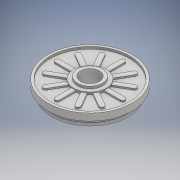
# Autodesk Inventor part: MotorGrill
Saved by Autodesk Inventor 2017 (Build 210142000, 142)
## iProperties
Created: 2017-08-24
Part Number: MotorGrill
Material: Generic
Document SubType Name: Modeling
Designer: MineV
Density: 1 g/cm^3
Appearance: Default
Author: MineV
Autodesk Inventor part; units mm, degrees
ref_plane "YZ Plane" through (0, 0, 0) normal (1, 0, 0) x (0, 1, 0)
ref_plane "XZ Plane" through (0, 0, 0) normal (0, 1, 0) x (-1, 0, 0)
ref_plane "XY Plane" through (0, 0, 0) normal (0, 0, 1) x (1, 0, 0)
sketch "Sketch1" plane through (0, 0, 0) normal (0, 1, 0) x (-1, 0, 0)
  line L0 (0, 0) -> (-27, 0)
  line L1 (-27, 0) -> (-27, -3)
  line L2 (-27, -3) -> (-22.5, -3)
  line L3 (-22.5, -3) -> (-22.5, -5.5)
  line L4 (-22.5, -5.5) -> (-24.5, -5.5)
  line L5 (-24.5, -5.5) -> (-24.5, -7.5)
  line L6 (-24.5, -7.5) -> (-20.5, -7.5)
  line L7 (-20.5, -7.5) -> (-20.5, -1.5)
  line L8 (-20.5, -1.5) -> (-8, -1.5)
  line L9 (-8, -1.5) -> (-8, -12.5)
  line L10 (-8, -12.5) -> (-6, -12.5)
  line L11 (-6, -12.5) -> (-6, 0)
  line L12 (-6, 0) -> (-6, 3)
  line L13 (-6, 3) -> (-8, 3)
  line L14 (-8, 3) -> (-8, 1.5)
  line L15 (-8, 1.5) -> (-9, 1.5)
  line L16 (-9, 1.5) -> (-10.5, 1.5)
  line L17 (-10.5, 1.5) -> (-10.5, 0)
  line L18 (-27, 0) -> (-27, 1.5)
  line L19 (-27, 1.5) -> (-25.5, 1.5)
  line L20 (-25.5, 1.5) -> (-25.5, 0)
  line L21 (0, -15.6) -> (0, 6.1) projected
  dimension "d0" = 27
  dimension "d1" = 3
  dimension "d2" = 4.5
  dimension "d3" = 2.5
  dimension "d4" = 2
  dimension "d5" = 2.5
  dimension "d6" = 4
  dimension "d7" = 2
  dimension "d8" = 1.5
  dimension "d9" = 8
  dimension "d10" = 3
  dimension "d11" = 2
  dimension "d12" = 1.5
  dimension "d13" = 1
  dimension "d14" = 1.5
  dimension "d15" = 1.5
  dimension "d16" = 5
  constraints: 42 end point, 14 perpendicular, 6 point on line, 2 horizontal, 2 vertical, 1 parallel
  measures "d0" distance of L0.start L0.end
  measures "d1" distance of L0.end L1.end
  measures "d2" distance of L1.end L2.end
  measures "d3" distance of L2.end L3.end
  measures "d4" distance of L4.end L5.end
  measures "d5" distance between parallel lines of L1 L5
  measures "d6" distance of L5.end L6.end
  measures "d7" distance of L9.end L10.end
  measures "d8" distance between parallel lines of L0 L8
  measures "d9" distance from line of L0.start L9
  measures "d10" distance of L11.end L12.end
  measures "d11" distance of L12.end L13.end
  measures "d12" distance of L13.end L14.end
  measures "d13" distance of L14.end L15.end
  measures "d14" distance of L15.end L16.end
  measures "d15" distance of L18.end L19.end
  measures "d16" distance between parallel lines of L6 L10
revolve "Revolution1" add sketch "Sketch1" angle 360 about axis through (0, 0, -10) along (0, 0, 1)
sketch "Sketch2" plane through (0, 0, 0) normal (0, 0, 1) x (1, 0, 0)
  circle A0 centre (0, 0) radius 10.5 projected
  line L0 (9.5, 1.5) -> (21, 1.5)
  line L1 (22.5, 0) -> (22.5, 0)
  line L2 (21, -1.5) -> (9.5, -1.5)
  line L3 (9.5, -1.5) -> (9.5, 1.5)
  arc A1 (22.5, 0) -> (21, 1.5) centre (21, 0) ccw
  arc A2 (21, -1.5) -> (22.5, 0) centre (21, 0) ccw
  line L4 (7.4772, 6.049) -> (17.4365, 11.799)
  line L5 (19.4856, 11.25) -> (19.4856, 11.25)
  line L6 (18.9365, 9.201) -> (8.9772, 3.451)
  line L7 (8.9772, 3.451) -> (7.4772, 6.049)
  arc A3 (19.4856, 11.25) -> (17.4365, 11.799) centre (18.1865, 10.5) ccw
  arc A4 (18.9365, 9.201) -> (19.4856, 11.25) centre (18.1865, 10.5) ccw
  line L8 (3.451, 8.9772) -> (9.201, 18.9365)
  line L9 (11.25, 19.4856) -> (11.25, 19.4856)
  line L10 (11.799, 17.4365) -> (6.049, 7.4772)
  line L11 (6.049, 7.4772) -> (3.451, 8.9772)
  arc A5 (11.25, 19.4856) -> (9.201, 18.9365) centre (10.5, 18.1865) ccw
  arc A6 (11.799, 17.4365) -> (11.25, 19.4856) centre (10.5, 18.1865) ccw
  line L12 (-1.5, 9.5) -> (-1.5, 21)
  line L13 (0, 22.5) -> (0, 22.5)
  line L14 (1.5, 21) -> (1.5, 9.5)
  line L15 (1.5, 9.5) -> (-1.5, 9.5)
  arc A7 (0, 22.5) -> (-1.5, 21) centre (0, 21) ccw
  arc A8 (1.5, 21) -> (0, 22.5) centre (0, 21) ccw
  line L16 (-6.049, 7.4772) -> (-11.799, 17.4365)
  line L17 (-11.25, 19.4856) -> (-11.25, 19.4856)
  line L18 (-9.201, 18.9365) -> (-3.451, 8.9772)
  line L19 (-3.451, 8.9772) -> (-6.049, 7.4772)
  arc A9 (-11.25, 19.4856) -> (-11.799, 17.4365) centre (-10.5, 18.1865) ccw
  arc A10 (-9.201, 18.9365) -> (-11.25, 19.4856) centre (-10.5, 18.1865) ccw
  line L20 (-8.9772, 3.451) -> (-18.9365, 9.201)
  line L21 (-19.4856, 11.25) -> (-19.4856, 11.25)
  line L22 (-17.4365, 11.799) -> (-7.4772, 6.049)
  line L23 (-7.4772, 6.049) -> (-8.9772, 3.451)
  arc A11 (-19.4856, 11.25) -> (-18.9365, 9.201) centre (-18.1865, 10.5) ccw
  arc A12 (-17.4365, 11.799) -> (-19.4856, 11.25) centre (-18.1865, 10.5) ccw
  line L24 (-9.5, -1.5) -> (-21, -1.5)
  line L25 (-22.5, 0) -> (-22.5, 0)
  line L26 (-21, 1.5) -> (-9.5, 1.5)
  line L27 (-9.5, 1.5) -> (-9.5, -1.5)
  arc A13 (-22.5, 0) -> (-21, -1.5) centre (-21, 0) ccw
  arc A14 (-21, 1.5) -> (-22.5, 0) centre (-21, 0) ccw
  line L28 (-7.4772, -6.049) -> (-17.4365, -11.799)
  line L29 (-19.4856, -11.25) -> (-19.4856, -11.25)
  line L30 (-18.9365, -9.201) -> (-8.9772, -3.451)
  line L31 (-8.9772, -3.451) -> (-7.4772, -6.049)
  arc A15 (-19.4856, -11.25) -> (-17.4365, -11.799) centre (-18.1865, -10.5) ccw
  arc A16 (-18.9365, -9.201) -> (-19.4856, -11.25) centre (-18.1865, -10.5) ccw
  line L32 (-3.451, -8.9772) -> (-9.201, -18.9365)
  line L33 (-11.25, -19.4856) -> (-11.25, -19.4856)
  line L34 (-11.799, -17.4365) -> (-6.049, -7.4772)
  line L35 (-6.049, -7.4772) -> (-3.451, -8.9772)
  arc A17 (-11.25, -19.4856) -> (-9.201, -18.9365) centre (-10.5, -18.1865) ccw
  arc A18 (-11.799, -17.4365) -> (-11.25, -19.4856) centre (-10.5, -18.1865) ccw
  line L36 (1.5, -9.5) -> (1.5, -21)
  line L37 (0, -22.5) -> (0, -22.5)
  line L38 (-1.5, -21) -> (-1.5, -9.5)
  line L39 (-1.5, -9.5) -> (1.5, -9.5)
  arc A19 (0, -22.5) -> (1.5, -21) centre (0, -21) ccw
  arc A20 (-1.5, -21) -> (0, -22.5) centre (0, -21) ccw
  line L40 (6.049, -7.4772) -> (11.799, -17.4365)
  line L41 (11.25, -19.4856) -> (11.25, -19.4856)
  line L42 (9.201, -18.9365) -> (3.451, -8.9772)
  line L43 (3.451, -8.9772) -> (6.049, -7.4772)
  arc A21 (11.25, -19.4856) -> (11.799, -17.4365) centre (10.5, -18.1865) ccw
  arc A22 (9.201, -18.9365) -> (11.25, -19.4856) centre (10.5, -18.1865) ccw
  line L44 (8.9772, -3.451) -> (18.9365, -9.201)
  line L45 (19.4856, -11.25) -> (19.4856, -11.25)
  line L46 (17.4365, -11.799) -> (7.4772, -6.049)
  line L47 (7.4772, -6.049) -> (8.9772, -3.451)
  arc A23 (19.4856, -11.25) -> (18.9365, -9.201) centre (18.1865, -10.5) ccw
  arc A24 (17.4365, -11.799) -> (19.4856, -11.25) centre (18.1865, -10.5) ccw
  point P0 (22.5, -1.5)
  point P1 (20.2356, 9.951)
  point P2 (12.549, 18.7356)
  point P3 (1.5, 22.5)
  point P4 (-9.951, 20.2356)
  point P5 (-18.7356, 12.549)
  point P6 (-22.5, 1.5)
  point P7 (-20.2356, -9.951)
  point P8 (-12.549, -18.7356)
  point P9 (-1.5, -22.5)
  point P10 (9.951, -20.2356)
  point P11 (18.7356, -12.549)
  dimension "d18" = 13
  dimension "d19" = 1
  dimension "d20" = 3
  dimension "d21" = 1.5
  dimension "d22" = 1.5
  dimension "d25" = 360
  constraints: 96 end point, 48 point on circle, 24 centre point, 24 point on line, 4 tangent, 2 parallel, 1 concentric, 1 horizontal, 1 perpendicular, 181 other
  measures "d18" distance of point (22.5, -1.5) L2.end
  measures "d19" distance edge to line of A0 L3
  measures "d20" distance of L2.end L0.start
  measures "d21" distance from line of point (0, 0) L0
  measures "d22" radius of A1
extrude "Extrusion1" add sketch "Sketch2" along normal blind 1 contours A0 L2 L3 L0 | A0 L0 A1 A2 L2 | L6 L7 L4 A0 | A0 L4 A3 A4 L6 | L44 A23 A24 L46 A0 | A0 L46 L47 L44 | L10 L11 L8 A0 | A0 L8 A5 A6 L10 | L40 A21 A22 L42 A0 | A0 L42 L43 L40 | L14 L15 L12 A0 | A0 L12 A7 A8 L14 | L36 A19 A20 L38 A0 | A0 L38 L39 L36 | L18 L19 L16 A0 | A0 L16 A9 A10 L18 | L32 A17 A18 L34 A0 | A0 L34 L35 L32 | L22 L23 L20 A0 | A0 L20 A11 A12 L22 | L28 A15 A16 L30 A0 | A0 L30 L31 L28 | L26 L27 L24 A0 | A0 L24 A13 A14 L26
sketch "Sketch3" plane through (0, 0, 0) normal (0, 1, 0) x (-1, 0, 0)
  line L0 (24.5, -5.5) -> (-24.5, -5.5) projected
  line L1 (22.4583, -5.5) -> (24.4583, -5.5)
  line L2 (24.4583, -5.5) -> (24.4583, -3)
  line L3 (24.4583, -3) -> (22.4583, -3)
  line L4 (22.4583, -3) -> (22.4583, -5.5)
  point P0 (0, 0)
  dimension "d29" = 2
  dimension "d30" = 2.5
  constraints: 8 end point, 2 parallel, 1 horizontal, 1 perpendicular, 1 point on line
  measures "d29" distance of L3.end L2.end
  measures "d30" distance of L2.end L1.end
extrude "Extrusion2" add sketch "Sketch3" against normal blind 1
equation "\"d21\" = 0.5 * d20"
body "Solid1"
